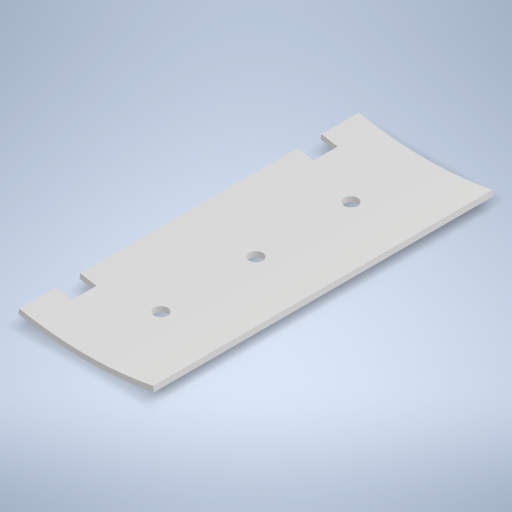
# Autodesk Inventor part: 214
Saved by Autodesk Inventor 2024 (Build 280153000, 153)
## iProperties
Created: 2024-06-10
Part Number: 214
Material: Generisch
Document SubType Name: Modeling
Designer: ffogue
Density: 1 g/cm^3
Appearance: Vorgabe
Author: ffogue
Autodesk Inventor part; units mm, degrees
ref_plane "YZ Plane" through (0, 0, 0) normal (1, 0, 0) x (0, 1, 0)
ref_plane "XZ Plane" through (0, 0, 0) normal (0, 1, 0) x (-1, 0, 0)
sketch "Skizze1" plane through (0, 0, 0) normal (0, 1, 0) x (-1, 0, 0)
  arc A0 (-19.7068, -62.5486) -> (19.7068, -62.5486) centre (0, 37) ccw
  line L0 (19.7068, -62.5486) -> (20, -64)
  arc A1 (-20, -64) -> (20, -64) centre (0, 35) ccw
  line L1 (-20, -64) -> (-19.7068, -62.5486)
  line L2 (0, -64.4804) -> (0, 0) construction
  point P0 (0, -64.4804)
  dimension "d0" = 2
  dimension "d1" = 101
  dimension "d2" = 40
  dimension "d3" = 35
  constraints: 6 end point, 6 point on circle, 3 vertical alignment, 2 centre point, 2 symmetric about line, 1 point on line, 1 vertical
  measures "d0" distance of A1.centre A0.centre
  measures "d1" radius of A1
  measures "d2" distance of L1.start L0.end
  measures "d3" distance of L2.end A1.centre
extrude "Extrusion1" add sketch "Skizze1" along normal blind 100
ref_plane "Arbeitsebene1" through (0, 0, -66) normal (0, 0, 1) x (1, 0, 0)
sketch "Skizze2" plane through (0, 0, -66) normal (0, 0, 1) x (1, 0, 0)
  line L0 (20, 100) -> (-20, 100) projected
  point P0 (0, 0)
  point P1 (0, 78)
  point P2 (0, 50)
  point P3 (0, 22)
  dimension "d7" = 22
  dimension "d8" = 22
  dimension "d9" = 28
  constraints: 3 vertical alignment
  measures "d7" distance from line of L0 point (0, 78)
  measures "d8" distance of point (0, 0) point (0, 22)
  measures "d9" distance of point (0, 50) point (0, 78)
hole "Bohrung1" at (0, 78, -66) at (0, 50, -66) at (0, 22, -66) direction (0, 0, 1) diameter 4 end through all
sketch "Skizze3" plane through (0, 0, -66) normal (0, 0, 1) x (1, 0, 0)
  line L0 (-20, 0) -> (-20, 100) projected
  line L1 (-20, 89) -> (-15, 89)
  line L2 (-15, 89) -> (-15, 82)
  line L3 (-15, 82) -> (-20, 82)
  line L4 (20, 100) -> (-20, 100) projected
  line L5 (-20, 11) -> (-15, 11)
  line L6 (-15, 11) -> (-15, 18)
  line L7 (-15, 18) -> (-20, 18)
  line L8 (20, 0) -> (-20, 0) projected
  point P0 (0, 0)
  point P1 (-17.5, 82)
  point P2 (-17.5, 89)
  dimension "d17" = 5
  dimension "d18" = 7
  dimension "d19" = 11
  dimension "d20" = 5
  dimension "d21" = 7
  dimension "d22" = 11
  constraints: 12 end point, 4 perpendicular, 4 point on line, 2 horizontal, 2 midpoint
  measures "d17" distance between parallel lines of L2 L0
  measures "d18" distance from line of point (-17.5, 82) L1
  measures "d19" distance from line of point (-17.5, 89) L4
  measures "d20" distance of L6.end L7.end
  measures "d21" distance between parallel lines of L5 L7
  measures "d22" distance between parallel lines of L8 L5
extrude "Extrusion2" cut sketch "Skizze3" along normal through all
